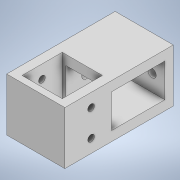
# Autodesk Inventor part: loacell_mount1
Saved by Autodesk Inventor 2022.3 (Build 263350000, 350)
## iProperties
Created: 2022-06-09
Part Number: loacell_mount1
Material: Generic
Document SubType Name: Modeling
Designer: Martijn
Density: 1 g/cm^3
Appearance: Default
Author: Martijn
Autodesk Inventor part; units mm, degrees
ref_plane "YZ Plane" through (0, 0, 0) normal (1, 0, 0) x (0, 1, 0)
ref_plane "XZ Plane" through (0, 0, 0) normal (0, 1, 0) x (-1, 0, 0)
ref_plane "XY Plane" through (0, 0, 0) normal (0, 0, 1) x (1, 0, 0)
sketch "Sketch1" plane through (0, 0, 0) normal (0, 0, 1) x (1, 0, 0)
  line L0 (0, 0) -> (44, 0)
  line L1 (44, 0) -> (44, 40)
  line L2 (44, 40) -> (0, 40)
  line L3 (0, 40) -> (0, 0)
  dimension "d0" = 44
  dimension "d1" = 40
  constraints: 8 end point, 2 parallel, 1 horizontal, 1 perpendicular
  measures "d0" distance of L0.start L0.end
  measures "d1" distance of L2.end L0.start
extrude "Extrusion1" add sketch "Sketch1" along normal blind 82
sketch "Sketch2" plane through (0, 0, 0) normal (0, -1, 0) x (1, 0, 0)
  line L0 (6.8, 77.2) -> (37.2, 77.2)
  line L1 (37.2, 77.2) -> (37.2, 46.8)
  line L2 (37.2, 46.8) -> (6.8, 46.8)
  line L3 (6.8, 46.8) -> (6.8, 77.2)
  line L4 (0, 0) -> (0, 82) projected
  line L5 (0, 82) -> (44, 82) projected
  dimension "d4" = 30.4
  dimension "d5" = 30.4
  dimension "d6" = 6.8
  dimension "d7" = 4.8
  constraints: 8 end point, 2 parallel, 1 horizontal, 1 perpendicular
  measures "d4" distance of L0.start L0.end
  measures "d5" distance of L2.end L0.start
  measures "d6" distance between parallel lines of L4 L3
  measures "d7" distance between parallel lines of L5 L0
extrude "Extrusion2" cut sketch "Sketch2" against normal blind 50
sketch "Sketch4" plane through (44, 0, 0) normal (1, 0, 0) x (0, 0, -1)
  line L0 (-6.4, 7.3) -> (-46.8, 7.3)
  line L1 (-46.8, 7.3) -> (-46.8, 32.7)
  line L2 (-46.8, 32.7) -> (-6.4, 32.7)
  line L3 (-6.4, 32.7) -> (-6.4, 7.3)
  line L4 (0, 0) -> (0, 40) projected
  line L5 (0, 0) -> (-82, 0) projected
  line L6 (-46.8, 0) -> (-46.8, 40) projected
  point P0 (0, 20)
  point P1 (-6.4, 20)
  dimension "d10" = 25.4
  dimension "d11" = 40.4
  dimension "d13" = 7.3
  constraints: 8 end point, 2 midpoint, 2 parallel, 1 collinear, 1 horizontal, 1 perpendicular
  measures "d10" distance between parallel lines of L0 L2
  measures "d11" distance between parallel lines of L3 L1
  measures "d13" distance between parallel lines of L5 L0
extrude "Extrusion3" cut sketch "Sketch4" against normal blind 34.4
sketch "Sketch6" plane through (44, 0, 0) normal (1, 0, 0) x (0, 0, -1)
  circle A0 centre (-62.2, 30) radius 2.5
  circle A1 centre (-62.2, 10) radius 2.5
  line L0 (0, 40) -> (-82, 40) projected
  line L1 (0, 0) -> (-82, 0) projected
  point P0 (-77.2, 40)
  dimension "d24" = 5
  dimension "d25" = 10
  dimension "d26" = 5
  dimension "d27" = 10
  dimension "d28" = 15
  dimension "d29" = 15
  constraints: 2 centre point
  measures "d24" diameter of A0
  measures "d25" distance from line of L0 A0.centre
  measures "d26" diameter of A1
  measures "d27" distance from line of L1 A1.centre
  measures "d28" horizontal distance of point (-77.2, 40) A1.centre
  measures "d29" horizontal distance of point (-77.2, 40) A0.centre
extrude "Extrusion5" cut sketch "Sketch6" against normal blind 50
sketch "Sketch5" plane through (0, 0, 0) normal (0, 0, -1) x (-1, 0, 0)
  circle A0 centre (-15.4, 20) radius 3.1
  circle A1 centre (-34.4, 20) radius 3.1
  line L0 (-44, 40) -> (0, 40) projected
  line L1 (-9.6, 7.3) -> (-9.6, 32.7) projected
  point P0 (0, 0)
  dimension "d16" = 6.2
  dimension "d17" = 6.2
  dimension "d18" = 20
  dimension "d19" = 20
  dimension "d20" = 5.8
  dimension "d21" = 19
  constraints: 2 centre point
  measures "d16" diameter of A0
  measures "d17" diameter of A1
  measures "d18" distance from line of L0 A0.centre
  measures "d19" distance from line of L0 A1.centre
  measures "d20" distance from line of L1 A0.centre
  measures "d21" distance of A0.centre A1.centre
extrude "Extrusion4" cut sketch "Sketch5" against normal blind 34
sketch "Sketch7" plane through (9.6, 0, 0) normal (1, 0, 0) x (0, 0, -1)
  circle A0 centre (-31.4, 19.8) radius 3.5
  line L0 (-6.4, 32.7) -> (-6.4, 7.3) projected
  line L1 (-6.4, 7.3) -> (-46.8, 7.3) projected
  point P0 (0, 0)
  dimension "d32" = 7
  dimension "d33" = 25
  dimension "d34" = 12.5
  constraints: 1 centre point
  measures "d32" diameter of A0
  measures "d33" distance from line of L0 A0.centre
  measures "d34" distance from line of L1 A0.centre
extrude "Extrusion6" cut sketch "Sketch7" against normal blind 34.4
body "Solid1"
